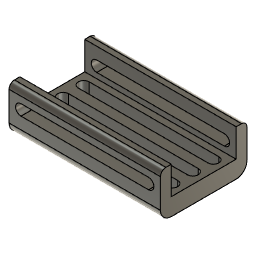
rtl-sdr-support (Autodesk Fusion 360 design; units mm, degrees)
Autodesk Fusion 360 part; units mm, degrees
sketch "Sketch1" plane through (0, 0, 0) normal (1, 0, 0) x (0, 1, 0)
  line L0 (0, 0) -> (0, 21)
  line L1 (0, 21) -> (5, 21)
  line L2 (5, 21) -> (5, 8)
  line L3 (5, 8) -> (35, 8)
  line L4 (35, 8) -> (35, 21)
  line L5 (35, 21) -> (40, 21)
  line L6 (40, 21) -> (40, 0)
  line L7 (40, 0) -> (0, 0)
  line L8 (20, 8) -> (20, 0) construction
  dimension "d1" = 8
  dimension "d2" = 30
  dimension "d3" = 5
  dimension "d5" = 5
  dimension "d6" = 13
  dimension "d7" = 13
  constraint coincident L0.start L7.end
  constraint vertical L0
  constraint perpendicular L0 L1
  constraint perpendicular L1 L2
  constraint perpendicular L2 L3
  constraint perpendicular L3 L4
  constraint perpendicular L2 L5
  constraint perpendicular L5 L6
  constraint perpendicular L0 L7
  constraint midpoint L3 L8.start
  constraint midpoint L7 L8.end
  measures "d1" distance of L3 L7
  measures "d2" distance of L2 L4
  measures "d3" distance of L0 L2
  measures "d5" distance of L4 L6
  measures "d6" distance of L1.end L2.end
  measures "d7" distance of L3.end L4.end
extrude "Extrude1" add sketch "Sketch1" along normal blind 70
fillet "Fillet1" radius 2.5 2 edges at (35, 40, 21) (35, 0, 21)
sketch "Sketch2" plane through (0, 0, 8) normal (0, 0, 1) x (-1, 0, 0)
  line L0 (0, -35) -> (0, -5)
  line L1 (0, -5) -> (-70, -5)
  line L2 (-70, -5) -> (-70, -35)
  line L3 (-70, -35) -> (0, -35)
  line L4 (0, -5) -> (-70, -5)
  line L5 (-70, -35) -> (-70, -5)
  line L6 (0, -5) -> (0, -35)
  line L7 (0, -35) -> (-70, -35)
  line L8 (-35, -35) -> (-35, -5) construction
  line L9 (-65, -10) -> (-65, -30) construction
  line L10 (-65, -30) -> (-5, -30) construction
  line L11 (-5, -30) -> (-5, -10) construction
  line L12 (-5, -10) -> (-65, -10) construction
  line L13 (-5, -20) -> (-65, -20) construction
  line L14 (-5, -27) -> (-65, -27)
  arc A0 (-65, -27) -> (-65, -32) centre (-65, -29.5) ccw
  line L15 (-65, -32) -> (-5, -32)
  arc A1 (-5, -32) -> (-5, -27) centre (-5, -29.5) ccw
  line L16 (-5, -29.5) -> (-65, -29.5) construction
  line L17 (-65, -22.5) -> (-5, -22.5)
  arc A2 (-5, -22.5) -> (-5, -17.5) centre (-5, -20) ccw
  line L18 (-5, -17.5) -> (-65, -17.5)
  arc A3 (-65, -17.5) -> (-65, -22.5) centre (-65, -20) ccw
  line L19 (-65, -13) -> (-5, -13)
  arc A4 (-5, -13) -> (-5, -8) centre (-5, -10.5) ccw
  line L20 (-5, -8) -> (-65, -8)
  arc A5 (-65, -8) -> (-65, -13) centre (-65, -10.5) ccw
  dimension "d12" = -5
  dimension "d15" = 3
  dimension "d16" = 5
  dimension "d19" = 0
  dimension "d20" = 19
  constraint midpoint L7 L8.start
  constraint midpoint L4 L8.end
  constraint midpoint L11 L13.start
  constraint midpoint L9 L13.end
  constraint tangent L14 A0
  constraint tangent A0 L15
  constraint parallel L14 L15
  constraint tangent L15 A1
  constraint tangent L14 A1
  constraint coincident L9 A0.centre
  constraint perpendicular L9 L16
  constraint coincident L11 A1.centre
  measures "d15" distance of L3 L15
  measures "d16" distance of L14 L15
extrude "Extrude2" cut sketch "Sketch2" against normal up to surface (8 mm away) contours L14 A0 L15 A1 | L17 A2 L18 A3 | L19 A4 L20 A5
sketch "Sketch3" plane through (0, 0, 0) normal (0, -1, 0) x (1, 0, 0)
  line L0 (70, 18.5) -> (0, 18.5)
  line L1 (0, 18.5) -> (0, 0)
  line L2 (0, 0) -> (70, 0)
  line L3 (70, 0) -> (70, 18.5)
  line L4 (0, 8) -> (70, 8)
  line L5 (0, 21) -> (70, 21)
  line L6 (0, 21) -> (0, 8)
  line L7 (70, 8) -> (70, 21)
  line L8 (0, 18.5) -> (70, 18.5)
  line L9 (5.5, 10.5) -> (64.5, 10.5)
  arc A0 (64.5, 10.5) -> (64.5, 15.5) centre (64.5, 13) ccw
  line L10 (64.5, 15.5) -> (5.5, 15.5)
  arc A1 (5.5, 15.5) -> (5.5, 10.5) centre (5.5, 13) ccw
  line L11 (5.5, 13) -> (64.5, 13) construction
  dimension "d23" = 5
  dimension "d24" = 3
  dimension "d25" = 3
  dimension "d26" = 3
  constraint tangent L9 A0
  constraint tangent A0 L10
  constraint parallel L9 L10
  constraint tangent L10 A1
  constraint tangent L9 A1
  constraint parallel L8 L11
  measures "d23" diameter of A0
  measures "d24" distance of L6 A1
  measures "d25" distance of L7 A0
  measures "d26" distance of L8 L10
extrude "Extrude3" cut sketch "Sketch3" against normal up to surface (40 mm away) contours L9 A0 L10 A1
fillet "Fillet2" radius 5 2 edges at (35, 40, 0) (35, 0, 0)
named bodies: "rtl-sdr-support"
